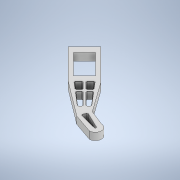
# Autodesk Inventor part: Lower_Limb
Saved by Autodesk Inventor 2021 (Build 250183000, 183)
## iProperties
Created: 2021-08-13
Part Number: Lower_Limb
Material: ABS Plastic
Document SubType Name: Modeling
Designer: rbnsmathew
Mass: 5.08543 g
Surface Area: 41.2479 cm^2
Volume: 4.79757 cm^3
Density: 1.06 g/cm^3
Appearance: Smooth - White
Author: rbnsmathew
Autodesk Inventor part; units mm, degrees
ref_plane "YZ Plane" through (0, 0, 0) normal (1, 0, 0) x (0, 1, 0)
ref_plane "XZ Plane" through (0, 0, 0) normal (0, 1, 0) x (-1, 0, 0)
ref_plane "XY Plane" through (0, 0, 0) normal (0, 0, 1) x (1, 0, 0)
sketch "Sketch1" plane through (0, 0, 0) normal (0, 1, 0) x (-1, 0, 0)
  line L0 (0, 0) -> (14.0954, -5.1303)
  line L1 (0, 0) -> (0, -5)
  line L2 (14.0954, -5.1303) -> (68.7081, -59.743)
  line L3 (0, 0) -> (53.7766, -44.8115)
  line L4 (0, 0) -> (0, 5)
  line L5 (14.0954, -5.1303) -> (15.8055, -0.4318)
  line L6 (14.0954, -5.1303) -> (12.3853, -9.8288)
  line L7 (0, 5) -> (15.8055, -0.4318)
  line L8 (0, -5) -> (12.3853, -9.8288)
  line L9 (36.8061, -37.0334) -> (53.4231, -53.6504)
  line L10 (53.4231, -53.6504) -> (62.6155, -44.458)
  line L11 (62.6155, -44.458) -> (45.9985, -27.841)
  line L12 (45.9985, -27.841) -> (36.8061, -37.0334)
  line L13 (36.8061, -37.0334) -> (62.6155, -44.458) construction
  line L14 (53.4231, -53.6504) -> (45.9985, -27.841) construction
  line L15 (30.2175, -34.8441) -> (55.4661, -60.0926)
  line L16 (55.4661, -60.0926) -> (68.9794, -46.5793)
  line L17 (68.9794, -46.5793) -> (44.0217, -21.6216)
  line L18 (37.7253, -28.7602) -> (36.2657, -30.2198)
  line L19 (30.2175, -34.8441) -> (68.9794, -46.5793) construction
  line L20 (55.4661, -60.0926) -> (44.0217, -21.6216) construction
  line L21 (15.8055, -0.4318) -> (44.0217, -21.6216)
  line L22 (12.3853, -9.8288) -> (30.2175, -34.8441)
  point P0 (49.7108, -40.7457)
  dimension "d10" = 15
  dimension "d11" = 70
  dimension "d12" = 155
  dimension "d13" = 70
  dimension "d14" = 5
  dimension "d15" = 5
  dimension "d16" = 5
  dimension "d17" = 5
  dimension "d18" = 6
  dimension "d19" = 13
  dimension "d20" = 23.5
  dimension "d21" = 6
  dimension "d22" = 3
  dimension "d23" = 56.1178
  constraints: 46 end point, 6 point on line, 4 parallel, 4 perpendicular, 2 midpoint, 2 vertical, 1 coincident
  measures "d10" distance of L0.start L0.end
  measures "d11" angle of L0 L1
  measures "d12" angle of L2 L0
  measures "d13" distance of L0.start L3.end
  measures "d14" distance of L0.start L4.end
  measures "d15" distance of L0.start L1.end
  measures "d16" distance of L0.end L5.end
  measures "d17" distance of L0.end L6.end
  measures "d18" distance from line of L10 L3.end
  measures "d19" distance between parallel lines of L9 L11
  measures "d20" distance between parallel lines of L10 L12
  measures "d21" distance between parallel lines of L16 L10
  measures "d22" distance between parallel lines of L17 L11
  measures "d23" distance of L0.end point (53.777, -44.812)
extrude "Extrusion1" add sketch "Sketch1" along normal blind 6 contours L4 L7 L5 L0 | L3 L8 L1 | L0 L6 L8 L3 | L5 L21 L17 L16 L2 L10 L11 L12 | L2 L18 L3 L22 L6 | L2 L12 L3 L18 | L3 L12 L9 L10 L2 L16 L15 L22
sketch "Sketch2" plane through (0, 0, 5) normal (1, 0, 0) x (0, 0, -1)
  line L0 (0, 0) -> (10, 0) projected
  line L1 (10, 0) -> (10, 6) projected
  line L2 (0, 6) -> (10, 6) projected
  line L3 (0, 0) -> (0, 6) projected
  line L4 (5, 6) -> (5, 0)
  constraints: 2 end point, 1 midpoint
revolve "Revolution1" add sketch "Sketch2" angle 180 about axis through (0, 6, 0) along (0, 1, 0) contours L3 L2 L4 L0
sketch "Sketch3" plane through (0, 6, 0) normal (0, 1, 0) x (1, 0, 0)
  line L0 (0, 5) -> (-12.3853, 9.8288) projected
  line L1 (-12.3853, 9.8288) -> (-30.2175, 34.8441) projected
  line L2 (-30.2175, 34.8441) -> (-55.4661, 60.0926) projected
  line L3 (-55.4661, 60.0926) -> (-68.9794, 46.5793) projected
  line L4 (-68.9794, 46.5793) -> (-44.0217, 21.6216) projected
  line L5 (-44.0217, 21.6216) -> (-15.8055, 0.4318) projected
  line L6 (-15.8055, 0.4318) -> (0, -5) projected
  arc A0 (0, -5) -> (0, 5) centre (0, 0) ccw projected
  line L7 (-36.8061, 37.0334) -> (-45.9985, 27.841) projected
  line L8 (-45.9985, 27.841) -> (-62.6155, 44.458) projected
  line L9 (-62.6155, 44.458) -> (-53.4231, 53.6504) projected
  line L10 (-53.4231, 53.6504) -> (-36.8061, 37.0334) projected
  line L11 (-44.0217, 21.6216) -> (-15.8055, 0.4318) projected
  line L12 (0, 0) -> (-14.0954, 5.1303)
  line L13 (-12.3853, 9.8288) -> (-30.2175, 34.8441) projected
  line L14 (-12.3853, 9.8288) -> (-15.8055, 0.4318)
  arc A1 (-0.1235, -0.4845) -> (0.2168, 0.4505) centre (0, 0) ccw
  line L15 (-14.0954, 5.1303) -> (-14.7794, 3.2509)
  line L16 (-14.0954, 5.1303) -> (-13.4113, 7.0097)
  line L17 (-14.7794, 3.2509) -> (-0.1235, -0.4845)
  line L18 (-13.4113, 7.0097) -> (0.2168, 0.4505)
  line L19 (-36.8061, 37.0334) -> (-45.9985, 27.841) projected
  line L20 (-41.4023, 32.4372) -> (-16.3159, 7.3508)
  line L21 (-36.8061, 37.0334) -> (-45.9985, 27.841) projected
  line L22 (-37.5132, 28.5481) -> (-33.2705, 32.7907)
  line L23 (-37.5132, 28.5481) -> (-41.7558, 24.3054)
  line L24 (-19.8355, 10.8704) -> (-22.6639, 8.042)
  line L25 (-19.8355, 10.8704) -> (-17.0071, 13.6988)
  line L26 (-17.0071, 13.6988) -> (-33.2705, 32.7907)
  line L27 (-22.6639, 8.042) -> (-41.7558, 24.3054)
  line L28 (-38.2203, 27.841) -> (-20.5426, 10.1633)
  line L29 (-19.1284, 11.5775) -> (-36.8061, 29.2552)
  line L30 (-27.8916, 26.4763) -> (-35.4414, 18.9265)
  line L31 (-33.914, 17.6254) -> (-26.5905, 24.9489)
  line L32 (-26.0922, 25.4497) -> (-34.877, 17.4267) construction
  line L33 (-34.4148, 17.1271) -> (-26.3917, 25.9119) construction
  line L34 (-30.4421, 21.477) -> (-34.1191, 17.8001)
  line L35 (-36.1498, 17.9923) -> (-36.176, 17.9662)
  point P0 (0, 0)
  point P1 (-30.9594, 23.4085)
  point P2 (-32.3736, 21.9943)
  point P3 (-30.9594, 20.5801)
  point P4 (-29.5452, 21.9943)
  dimension "d40" = 1
  dimension "d41" = 2
  dimension "d42" = 2
  dimension "d53" = 6
  dimension "d54" = 6
  dimension "d55" = 4
  dimension "d56" = 4
  dimension "d57" = 25
  dimension "d58" = 1
  dimension "d59" = 1
  dimension "d60" = 15
  dimension "d61" = 2
  dimension "d67" = 5.5
  constraints: 42 end point, 18 point on line, 7 parallel, 4 perpendicular, 2 coincident, 2 midpoint, 2 point on circle, 2 tangent, 1 centre point
  measures "d40" diameter of A1
  measures "d41" distance of L12.end L15.end
  measures "d42" distance of L12.end L16.end
  measures "d53" distance of L22.start L22.end
  measures "d54" distance of L22.start L23.end
  measures "d55" distance of L24.start L25.end
  measures "d56" distance of L24.start L24.end
  measures "d57" distance of L24.start L22.start
  measures "d58" distance between parallel lines of L20 L29
  measures "d59" distance between parallel lines of L28 L20
  measures "d60" distance of L24.start L34.start
  measures "d61" distance between parallel lines of L30 L31
  measures "d67" distance between parallel lines of L7 L22
extrude "Extrusion3" cut sketch "Sketch3" against normal blind 6 contours L18 A1 L17 L14 | L22 L26 L30 L29 | L28 L30 L27 L23 | L31 L26 L25 L29 | L28 L24 L27 L31
chamfer "Chamfer3" distance 0.75 angle 45 18 edges at (-41.7558, 3, -24.3054) (-36.8061, 3, -29.2552) (-33.914, 3, -17.6254) (-29.5452, 3, -21.9943) (-33.2705, 3, -32.7907) (-38.2203, 3, -27.841) (-30.9594, 3, -20.5801) (-26.5905, 3, -24.9489) (-22.6639, 3, -8.042) (-35.4414, 3, -18.9265) (-30.9594, 3, -23.4085) (-19.1284, 3, -11.5775) (-32.3736, 3, -21.9943) (-20.5426, 3, -10.1633) (-17.0071, 3, -13.6988) (-27.8916, 3, -26.4763) (-14.7794, 3, -3.2509) (-13.4113, 3, -7.0097)
chamfer "Chamfer4" distance 0.25 angle 45 32 edges at (-30.581, 6, -29.6335) (-33.2925, 6, -32.2401) (-35.0383, 6, -31.023) (-36.2757, 6, -29.2552) (-33.8827, 6, -26.3318) (-30.9594, 6, -23.9388) (-29.4255, 6, -24.9424) (-28.3999, 6, -26.4966) (-39.988, 6, -26.0732) (-38.2203, 6, -27.3106) (-35.2969, 6, -24.9176) (-32.9039, 6, -21.9943) (-33.9075, 6, -20.4604) (-35.4617, 6, -19.4348) (-38.5986, 6, -21.616) (-41.2052, 6, -24.3274) (-28.0678, 6, -23.4716) (-29.0148, 6, -21.9943) (-24.3368, 6, -16.7859) (-26.6125, 6, -24.3983) (-21.7988, 6, -19.3239) (-32.4367, 6, -19.1027) (-30.9594, 6, -20.0497) (-25.751, 6, -15.3717) (-33.3634, 6, -17.6474) (-28.289, 6, -12.8337) (-22.6842, 6, -8.5503) (-21.6033, 6, -9.1026) (-21.0729, 6, -10.1633) (-19.1284, 6, -12.1079) (-18.0677, 6, -12.6382) (-17.5154, 6, -13.7191)
chamfer "Chamfer5" distance 0.25 angle 45 42 edges at (-6.2594, 6, -3.5675) (-7.0881, 6, -1.2906) (-14.0954, 6, -5.1303) (-13.2017, 6, -6.4947) (-14.2878, 6, -3.5107) (-35.2969, 0, -24.9176) (-38.2203, 0, -27.3106) (-39.988, 0, -26.0732) (-41.2052, 0, -24.3274) (-38.5986, 0, -21.616) (-35.4617, 0, -19.4348) (-33.9075, 0, -20.4604) (-32.9039, 0, -21.9943) (-33.8827, 0, -26.3318) (-36.2757, 0, -29.2552) (-35.0383, 0, -31.023) (-33.2925, 0, -32.2401) (-30.581, 0, -29.6335) (-28.3999, 0, -26.4966) (-29.4255, 0, -24.9424) (-30.9594, 0, -23.9388) (-28.0678, 0, -23.4716) (-29.0148, 0, -21.9943) (-24.3368, 0, -16.7859) (-26.6125, 0, -24.3983) (-21.7988, 0, -19.3239) (-19.1284, 0, -12.1079) (-18.0677, 0, -12.6382) (-17.5154, 0, -13.7191) (-14.0954, 0, -5.1303) (-14.2878, 0, -3.5107) (-7.0881, 0, -1.2906) (-6.2594, 0, -3.5675) (-13.2017, 0, -6.4947) (-28.289, 0, -12.8337) (-33.3634, 0, -17.6474) (-32.4367, 0, -19.1027) (-30.9594, 0, -20.0497) (-25.751, 0, -15.3717) (-21.0729, 0, -10.1633) (-21.6033, 0, -9.1026) (-22.6842, 0, -8.5503)
equation "\"d15\" = d14"
equation "\"d17\" = d16"
equation "\"d42\" = d41"
equation "\"d54\" = d53"
equation "\"d56\" = d55"
equation "\"d59\" = d58"
body "Solid1"
